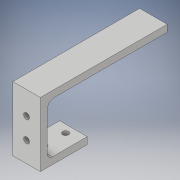
# Autodesk Inventor part: U bracket
Saved by Autodesk Inventor 2019 (Build 230136000, 136)
## iProperties
Created: 2020-10-22
Part Number: U bracket
Material: Generic
Document SubType Name: Modeling
Designer: Delta
Density: 1 g/cm^3
Appearance: Default
Author: Delta
Autodesk Inventor part; units mm, degrees
ref_plane "YZ Plane" through (0, 0, 0) normal (1, 0, 0) x (0, 1, 0)
ref_plane "XZ Plane" through (0, 0, 0) normal (0, 1, 0) x (-1, 0, 0)
ref_plane "XY Plane" through (0, 0, 0) normal (0, 0, 1) x (1, 0, 0)
sketch "Sketch1" plane through (0, 0, 0) normal (1, 0, 0) x (0, 1, 0)
  line L0 (0, 0) -> (3.175, 0)
  line L1 (3.175, 0) -> (3.175, -21.59)
  line L2 (3.175, -21.59) -> (0, -21.59)
  line L3 (0, -21.59) -> (0, 0)
  line L4 (0, 0) -> (29.591, 0)
  line L5 (29.591, 0) -> (29.591, -3.175)
  line L6 (29.591, -3.175) -> (0, -3.175)
  line L7 (0, -3.175) -> (0, 0)
  line L8 (29.591, 0) -> (26.416, 0)
  line L9 (26.416, 0) -> (26.416, -58.42)
  line L10 (26.416, -58.42) -> (29.591, -58.42)
  line L11 (29.591, -58.42) -> (29.591, 0)
  dimension "d0" = 3.175
  dimension "d1" = 21.59
  dimension "d4" = 3.175
  dimension "d5" = 29.591
  dimension "d6" = 3.175
  dimension "d7" = 58.42
  constraints: 24 end point, 6 parallel, 3 horizontal, 3 perpendicular
  measures "d0" distance of L1.end L2.end
  measures "d1" distance of L0.end L1.end
  measures "d4" distance of L9.end L10.end
  measures "d5" distance of L0.start L4.end
  measures "d6" distance between parallel lines of L4 L6
  measures "d7" distance of L10.end L4.end
extrude "Extrusion1" add sketch "Sketch1" along normal blind 12.7
sketch "Sketch2" plane through (0, 3.175, -3.175) normal (0, 0, -1) x (-1, 0, 0)
  circle A0 centre (-6.35, 15.8052) radius 1.3589
  circle A1 centre (-6.35, 6.1786) radius 1.3589
  line L0 (-12.7, 0) -> (-12.7, 23.241) projected
  point P0 (0, -3.175)
  dimension "d8" = 2.7178
  dimension "d9" = 2.7178
  dimension "d10" = 6.35
  dimension "d11" = 6.35
  dimension "d12" = 9.6266
  constraints: 2 centre point
  measures "d8" diameter of A0
  measures "d9" diameter of A1
  measures "d10" distance from line of L0 A0.centre
  measures "d11" distance from line of L0 A1.centre
  measures "d12" distance of A1.centre A0.centre
extrude "Extrusion2" cut sketch "Sketch2" against normal blind 25.4
sketch "Sketch3" plane through (0, 3.175, -3.175) normal (0, 1, 0) x (1, 0, 0)
  circle A0 centre (6.35, 4.8202) radius 1.3589
  circle A1 centre (6.35, 14.8278) radius 1.3589
  line L0 (0, 18.415) -> (0, 0) projected
  point P0 (0, -3.175)
  dimension "d15" = 2.7178
  dimension "d16" = 2.7178
  dimension "d17" = 6.35
  dimension "d18" = 6.35
  dimension "d23" = 10.0076
  constraints: 2 centre point
  measures "d15" diameter of A0
  measures "d16" diameter of A1
  measures "d17" distance from line of L0 A1.centre
  measures "d18" distance from line of L0 A0.centre
  measures "d23" distance of A1.centre A0.centre
extrude "Extrusion3" cut sketch "Sketch3" against normal blind 25.4
fillet "Fillet1" radius 3.175 1 edges at (6.35, 26.416, -3.175)
fillet "Fillet2" radius 2.286 1 edges at (6.35, 3.175, -3.175)
equation "\"d4\" = d0"
equation "\"d6\" = d0"
body "Solid1"
